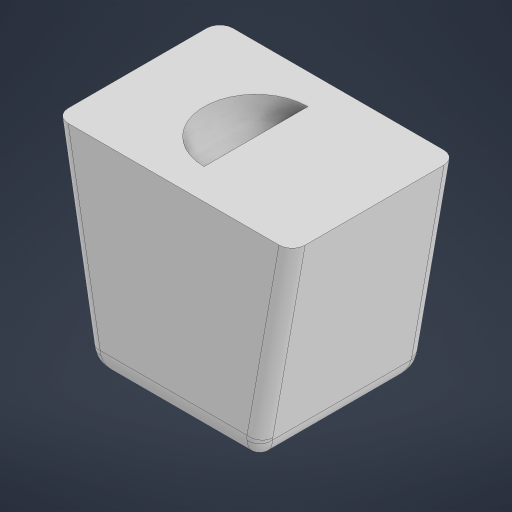
# Autodesk Inventor part: OwnSpectr_TubeHolder_D
Saved by Autodesk Inventor 2024.1 (Build 281209000, 209)
## iProperties
Created: 2024-08-12
Part Number: OwnSpectr_TubeHolder_D
Material: Generic
Document SubType Name: Modeling
Designer: Tim Jäger
Density: 1 g/cm^3
Appearance: Default
Author: Tim Jäger
## iProperties of the stored document OwnSpectr_TubeHolder_D_3DPrint.ipt
Created: 2024-08-16
Part Number: OwnSpectr_TubeHolder_D_3DPrint
Material: Generic
Document SubType Name: Modeling
Designer: Tim Jäger
Density: 1 g/cm^3
Appearance: Default
Author: Tim Jäger
Autodesk Inventor part; units mm, degrees
ref_plane "YZ Plane" through (0, 0, 0) normal (1, 0, 0) x (0, 1, 0)
ref_plane "XZ Plane" through (0, 0, 0) normal (0, 1, 0) x (-1, 0, 0)
ref_plane "XY Plane" through (0, 0, 0) normal (0, 0, 1) x (1, 0, 0)
sketch "Sketch1" plane through (0, 0, 0) normal (0, 0, 1) x (1, 0, 0)
  line L0 (-6.32, 0) -> (-9.14, 15.933)
  line L1 (-9.14, 15.933) -> (9.14, 15.933)
  line L2 (9.14, 15.933) -> (6.32, 0)
  line L3 (6.32, 0) -> (-6.32, 0)
  point P0 (0, 0)
  point P1 (0, 15.933)
  point P2 (0, 0)
  dimension "d0" = 2.82
  dimension "d1" = 15.933
  dimension "d2" = 12.64
  constraints: 8 end point, 2 horizontal, 2 midpoint, 2 vertical alignment, 1 equal length, 1 horizontal alignment
  measures "d0" horizontal distance of L0.start L0.end
  measures "d1" distance between parallel lines of L1 L3
  measures "d2" distance of L2.end L0.start
extrude "Extrusion1" add sketch "Sketch1" along normal blind 12.7
fillet "Fillet1" radius 2 4 edges at (0, 0, 0) (6.32, 0, 6.35) (0, 0, 12.7) (-6.32, 0, 6.35)
fillet "Fillet2" radius 1 12 edges at (7.907, 8.9665, 12.7) (5.928, 0.4675, 11.9851) (6.643, 1.825, 12.6923) (5.928, 0.4675, 0.7149) (7.907, 8.9665, 0) (6.643, 1.825, 0.0077) (-6.643, 1.825, 0.0077) (-7.907, 8.9665, 0) (-5.928, 0.4675, 0.7149) (-5.928, 0.4675, 11.9851) (-7.907, 8.9665, 12.7) (-6.643, 1.825, 12.6923)
sketch "Sketch2" plane through (-8.1245, 15.933, 0) normal (0, 1, 0) x (1, 0, 0)
  arc A0 (8.1245, -2.35) -> (8.1245, -10.35) centre (8.1245, -6.35) ccw
  line L0 (16.2489, 0) -> (0, 0) projected
  line L1 (8.1245, -10.35) -> (8.1245, -2.35)
  line L2 (-1.0155, -1) -> (-1.0155, -11.7) projected
  point P0 (8.1245, 0)
  point P1 (8.1245, 0)
  point P2 (-1.0155, -6.35)
  dimension "d7" = 4
  constraints: 3 midpoint, 3 vertical alignment, 2 end point, 2 point on circle, 1 centre point, 1 horizontal alignment, 1 vertical
  measures "d7" radius of A0
revolve "Revolution1" cut sketch "Sketch2" angle 135 about axis through (0, 15.933, 10.35) along (0, 0, 1)
body "Solid1"
